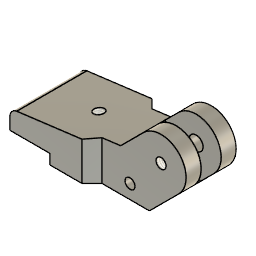
39 (Autodesk Fusion 360 design; units mm, degrees)
Autodesk Fusion 360 part; units mm, degrees
sketch "草图1" plane through (0, 0, 0) normal (0, 1, 0) x (1, 0, 0)
  line L0 (0, 0) -> (44.67767, 0)
  line L1 (44.67767, 0) -> (59.338835, -14.661165)
  arc A0 (41.661165, -32.338835) -> (59.338835, -14.661165) centre (50.5, -23.5) ccw
  line L2 (41.661165, -32.338835) -> (30.32233, -21)
  line L3 (30.32233, -21) -> (-16.50833, -15)
  arc A1 (-20, -11.032431) -> (-16.50833, -15) centre (-16, -11.032431) ccw
  line L4 (-20, -11.032431) -> (-20, -5)
  line L5 (-20, -5) -> (0, -5)
  line L6 (0, -5) -> (0, 0)
  circle A2 centre (35, -7) radius 2.5
  dimension "d1" = 5
  dimension "d2" = 20
  dimension "d3" = 4
  dimension "d4" = 135
  dimension "d5" = 35
  dimension "d6" = 12.5
  dimension "d7" = 23.5
  dimension "d8" = 70.5
  dimension "d9" = 5
  dimension "d10" = 7
  dimension "d11" = 21
  dimension "d12" = 10
  constraint coincident L0.start L6.end
  constraint horizontal L0
  constraint tangent L1 A0
  constraint parallel L1 L2
  constraint tangent L3 A1
  constraint vertical L4
  constraint perpendicular L4 L5
  constraint perpendicular L0 L6
  constraint tangent A1 L4
  constraint tangent A0 L2
  measures "d1" distance of L5.end L0.start
  measures "d2" horizontal distance of L0.start L4.end
  measures "d3" radius of A1
  measures "d4" angle of L0 L1
  measures "d5" horizontal distance of L0.start A2.centre
  measures "d6" radius of A0
  measures "d7" distance of L0 A0.centre
  measures "d8" horizontal distance of A0.centre L4.end
  measures "d9" diameter of A2
  measures "d10" distance of L0 A2.centre
extrude "拉伸1" add sketch "草图1" along normal blind 35 contours L0 L1 A0 L2 L3 A1 L4 L5 L6 picked at (45.852908, -18.651526)
sketch "草图2" plane through (0, 0, 0) normal (0, 0, 1) x (1, 0, 0)
  line L0 (-20, 0) -> (-20, 35)
  line L1 (-20, 35) -> (16, 35)
  line L2 (16, 35) -> (21, 30)
  line L3 (21, 30) -> (105, 30)
  line L4 (105, 30) -> (105, 5)
  line L5 (105, 5) -> (21, 5)
  line L6 (21, 5) -> (16, 0)
  line L7 (16, 0) -> (-20, 0)
  line L8 (-55, 0) -> (65, 0) construction
  line L9 (-20, 17.5) -> (-60, 17.5) construction
  dimension "d15" = 20
  dimension "d16" = 35
  dimension "d17" = 36
  dimension "d18" = 135
  dimension "d19" = 135
  dimension "d20" = 25
  dimension "d21" = 125
  constraint vertical L0
  constraint perpendicular L0 L1
  constraint perpendicular L0 L3
  constraint perpendicular L3 L4
  constraint perpendicular L0 L7
  constraint horizontal L8
  constraint collinear L7 L8
  constraint equal L1 L7
  constraint parallel L5 L8
  constraint midpoint L0 L9.start
  constraint perpendicular L4 L9
  constraint symmetric L3 L5 L9
  measures "d15" distance of origin L0.start
  measures "d16" distance of L0.start L0.end
  measures "d17" distance of L0.start L6.end
  measures "d18" angle of L6 L7
  measures "d19" angle of L1 L2
  measures "d20" distance of L3.end L4.end
  measures "d21" distance of L0 L4
extrude "拉伸2" cut sketch "草图2" along normal blind 85 contours L0 L1 L2 L3 L4 L5 L6 L7 picked at (77, 21.666667) keep common part
sketch "草图3" plane through (4.661165, 0, -4.661165) normal (-0.707107, 0, 0.707107) x (0, -1, 0)
  line L0 (-30, 52.325902) -> (-30, 36.290368)
  line L1 (-30, 36.290368) -> (-5, 36.290368)
  line L2 (-5, 36.290368) -> (-5, 52.325902)
  line L3 (-5, 52.325902) -> (-30, 52.325902)
  line L4 (-17.5, 36.290368) -> (-17.5, 72.000001) construction
  line L5 (-19.5, 39.825902) -> (-15.5, 39.825902)
  line L6 (-12.5, 39.825902) -> (-12.5, 64.825902)
  line L7 (-12.5, 64.825902) -> (-22.5, 64.825902)
  line L8 (-22.5, 64.825902) -> (-22.5, 42.825902)
  arc A0 (-15.5, 39.825902) -> (-12.5, 42.825902) centre (-12.5, 39.825902) ccw
  arc A1 (-22.5, 42.825902) -> (-19.5, 39.825902) centre (-22.5, 39.825902) ccw
  dimension "d24" = 6
  dimension "d25" = 10
  dimension "d26" = 12.5
  dimension "d27" = 25
  constraint equal A0 A1
  constraint perpendicular L1 L4
  constraint perpendicular L5 L6
  constraint perpendicular L6 L7
  constraint perpendicular L5 L8
  measures "d24" diameter of A1
extrude "拉伸3" cut sketch "草图3" against normal blind 61 contours L3 L6 L7 L8 | L3 L5 L6 L8 A0 A1 picked at (-15.833333, 56.492568) picked at (-19.166667, 49.159235)
sketch "草图4" plane through (0, 30, 0) normal (0, 1, 0) x (-1, 0, 0)
  line L0 (-21, 19.805612) -> (-30.32233, 21)
  line L1 (-30.32233, 21) -> (-41.661165, 32.338835)
  arc A0 (-41.661165, 32.338835) -> (-59.338835, 14.661165) centre (-50.5, 23.5) ccw
  line L2 (-59.338835, 14.661165) -> (-44.67767, 0)
  line L3 (-44.67767, 0) -> (-21, 0)
  line L4 (-21, 0) -> (-21, 19.805612)
  circle A1 centre (-35, 7) radius 2.5
  circle A2 centre (-50.5, 23.5) radius 3.5
  dimension "d30" = 7
  constraint concentric A0 A2
  measures "d30" diameter of A2
extrude "拉伸4" cut sketch "草图4" against normal blind 15 contours A2 picked at (-51.083333, 24.076707)
sketch "草图5" plane through (0, 5, 0) normal (0, -1, 0) x (1, 0, 0)
  line L0 (30.32233, 21) -> (21, 19.805612)
  line L1 (21, 19.805612) -> (21, 0)
  line L2 (21, 0) -> (44.67767, 0)
  line L3 (44.67767, 0) -> (59.338835, 14.661165)
  arc A0 (59.338835, 14.661165) -> (41.661165, 32.338835) centre (50.5, 23.5) ccw
  line L4 (41.661165, 32.338835) -> (30.32233, 21)
  circle A1 centre (35, 7) radius 2.5
hole "孔1" at (50.5, 5, 23.5) direction (0, 1, 0) diameter 6 depth 13 tip angle 180
thread "螺纹1" "ISO Metric profile 6.0 M6x1 M6x1 6H" major diameter 6.147 minor diameter 5.035 pitch 1 angle 60 resizes the face on face at (50.798704, 7.5, 26.485092)
sketch "草图6" plane through (0, 0, 0) normal (0, 0, -1) x (1, 0, 0)
  line L0 (16, -35) -> (21, -30)
  line L1 (21, -30) -> (44.67767, -30)
  line L2 (44.67767, -30) -> (44.67767, -5)
  line L3 (44.67767, -5) -> (21, -5)
  line L4 (21, -5) -> (16, 0)
  line L5 (16, 0) -> (0, 0)
  line L6 (0, 0) -> (0, -35)
  line L7 (0, -35) -> (16, -35)
  circle A0 centre (7, -17.5) radius 4.5
  dimension "d38" = 7
  dimension "d39" = 9
  dimension "d40" = 17.5
  measures "d38" distance of L6 A0.centre
  measures "d39" diameter of A0
  measures "d40" distance of L5 A0.centre
extrude "拉伸5" cut sketch "草图6" against normal blind 5 contours A0 picked at (6.233246, -18.575475)
sketch "草图7" plane through (0, 0, 5) normal (0, 0, -1) x (1, 0, 0)
  circle A0 centre (7, -17.5) radius 4.5
  circle A1 centre (7, -17.5) radius 3
  dimension "d43" = 6
  constraint concentric A0 A1
  measures "d43" diameter of A1
extrude "拉伸6" cut sketch "草图7" against normal blind 92 contours A1 picked at (5.87651, -18.041044)
thread "螺纹2" "ISO Metric profile 6.0 M6x1 M6x1 6H" major diameter 6.147 minor diameter 5.035 pitch 1 angle 60 resizes the face on face at (9.991104, 17.269137, 9.465001)
equation "d26 = 25 mm - 12.5 mm"
